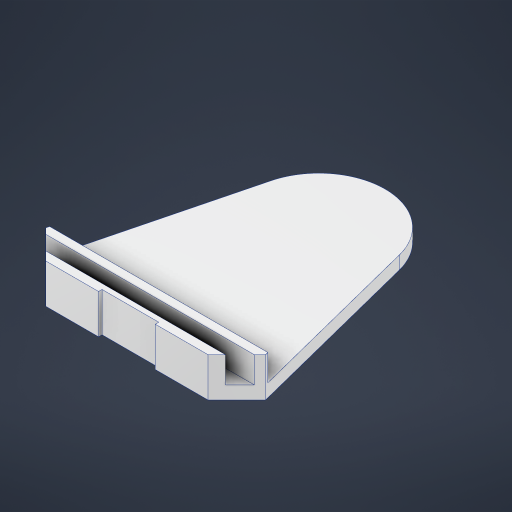
# Autodesk Inventor part: KrovatkaShatunFlanec
Saved by Autodesk Inventor 2024 (Build 280153000, 153)
## iProperties
Created: 2023-12-22
Part Number: KrovatkaShatunFlanec
Material: Aluminum 6061
Document SubType Name: Modeling
Designer: KirikDK
Mass: 2537.18 g
Surface Area: 1505.8 cm^2
Volume: 939.698 cm^3
Density: 2.7 g/cm^3
Appearance: Aluminum - Flat
Author: KirikDK
Autodesk Inventor part; units mm, degrees
ref_plane "YZ Plane" through (0, 0, 0) normal (1, 0, 0) x (0, 1, 0)
ref_plane "XZ Plane" through (0, 0, 0) normal (0, 1, 0) x (-1, 0, 0)
ref_plane "XY Plane" through (0, 0, 0) normal (0, 0, 1) x (1, 0, 0)
sketch "Sketch1" plane through (0, 0, 0) normal (0, 1, 0) x (-1, 0, 0)
  circle A0 centre (-6.6375, -88.2502) radius 58
  line L0 (-14.6375, 98.7498) -> (-14.6375, -12.6724)
  arc A1 (-14.6375, -12.6724) -> (-73.5777, -52.264) centre (-6.6375, -88.2502) ccw
  line L1 (-73.5777, -52.264) -> (-112.0003, 98.7498)
  line L2 (-112.0003, 98.7498) -> (-14.6375, 98.7498)
  line L3 (98.7253, 98.7498) -> (60.3027, -52.264)
  arc A2 (60.3027, -52.264) -> (1.3625, -12.6724) centre (-6.6375, -88.2502) ccw
  line L4 (1.3625, -12.6724) -> (1.3625, 98.7498)
  line L5 (1.3625, 98.7498) -> (98.7253, 98.7498)
  line L6 (67.0159, -106.9899) -> (119.3625, 98.7498)
  line L7 (119.3625, 98.7498) -> (119.3625, 131.7498)
  line L8 (119.3625, 131.7498) -> (-132.6375, 131.7498)
  line L9 (-132.6375, 131.7498) -> (-132.6375, 98.7498)
  line L10 (-132.6375, 98.7498) -> (-80.2909, -106.9899)
  arc A3 (-80.2909, -106.9899) -> (67.0159, -106.9899) centre (-6.6375, -88.2502) ccw
  constraints: 22 end point, 6 point on circle, 4 centre point
extrude "Extrusion1" add sketch "Sketch1" along normal blind 15 contours A0 | L0 A1 L1 L2 | L3 A2 L4 L5 | A3 L10 L9 L8 L7 L6
chamfer "Chamfer1" distance 33 angle 45 2 edges at (-119.3625, 7.5, 131.7498) (132.6375, 7.5, 131.7498)
sketch "Sketch4" plane through (0, 15, 0) normal (0, 1, 0) x (1, 0, 0)
  line L0 (132.6375, -98.7498) -> (99.6375, -131.7498) projected
  line L1 (132.6375, -98.7498) -> (80.2909, 106.9899) projected
  arc A0 (80.2909, 106.9899) -> (-67.0159, 106.9899) centre (6.6375, 88.2502) ccw projected
  line L2 (-67.0159, 106.9899) -> (-119.3625, -98.7498) projected
  line L3 (-86.3625, -131.7498) -> (-119.3625, -98.7498) projected
  line L4 (-86.3625, -131.7498) -> (99.6375, -131.7498) projected
  line L5 (-97.308, -131.7498) -> (123, -131.7498)
  line L6 (123, -131.7498) -> (123, -121.7498)
  line L7 (123, -121.7498) -> (-97.308, -121.7498)
  line L8 (-97.308, -121.7498) -> (-97.308, -131.7498)
  line L9 (-122.7338, -105.2498) -> (137.8877, -105.2498)
  line L10 (137.8877, -105.2498) -> (137.8877, -95.2498)
  line L11 (137.8877, -95.2498) -> (-122.7338, -95.2498)
  line L12 (-122.7338, -95.2498) -> (-122.7338, -105.2498)
  point P0 (0, 0)
  point P1 (109.6375, -121.7498)
  point P2 (-96.3625, -121.7498)
  point P3 (131.747, -95.2498)
  point P4 (-118.472, -95.2498)
  point P5 (-118.8536, -96.7498)
  point P6 (132.1287, -96.7498)
  point P7 (-112.8625, -105.2498)
  point P8 (126.1375, -105.2498)
  dimension "d5" = 10
  dimension "d6" = 10
  dimension "d7" = 16.5
  constraints: 16 end point, 4 parallel, 2 horizontal, 2 perpendicular, 1 point on line
  measures "d5" distance between parallel lines of L9 L11
  measures "d6" distance between parallel lines of L7 L4
  measures "d7" distance between parallel lines of L9 L7
extrude "Extrusion2" add sketch "Sketch4" along normal blind 30 contours L0 L9 L3 L2 L11 L1 | L0 L4 L3 L7
sketch "Sketch5" plane through (-86.3625, 0, 131.7498) normal (0, 0, 1) x (1, 0, 0)
  line L0 (196, 45) -> (-10, 45) projected
  line L1 (0, 0) -> (186, 0) projected
  line L2 (60.5, 45) -> (125.5, 45)
  line L3 (125.5, 45) -> (125.5, 0)
  line L4 (125.5, 0) -> (60.5, 0)
  line L5 (60.5, 0) -> (60.5, 45)
  line L6 (186, 45) -> (186, 0) projected
  line L7 (0, 0) -> (0, 45) projected
  point P0 (86.3625, 0)
  point P1 (186, 22.5)
  point P2 (0, 22.5)
  dimension "d10" = 65
  dimension "d11" = 60.5
  dimension "d12" = 60.5
  constraints: 8 end point, 2 midpoint, 2 parallel, 2 point on line, 1 horizontal, 1 perpendicular
  measures "d10" distance between parallel lines of L3 L5
  measures "d11" distance from line of point (186, 22.5) L3
  measures "d12" distance from line of L5 point (0, 22.5)
extrude "Extrusion3" cut sketch "Sketch5" against normal blind 4 contours L3 L1 L5 L0
body "Solid1"
